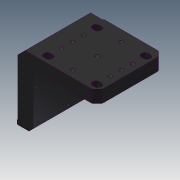
# Autodesk Inventor part: J003053
Saved by Autodesk Inventor 2015 SP1 (Build 190203100, 203)
## iProperties
Created: 2015-01-06
Material: ALUMINUM, 6061-T651
Vendor: HHMI: JFRC - ID&F
Document SubType Name: Modeling
Designer: ARNOLDJ
Density: 2.7 g/cm^3
Mass: 325.965 g
Surface Area: 259.814 cm^2
Volume: 120.728 cm^3
Description: MBS CONN LINK
Project: P-201804
Appearance: Rubber - Black
Part Number: J003053
RuleStatus: InUse
AfterDocSave0: file://Part Number Cleaner
LAB/DEPT: SVOBODA (LAB)
REQUESTING SCIENTIST: SOFRONIEW, NICK
SURFACE ROUGHNESS: 63 Ra
DESIGN DEPARTMENT: HHMI: JRC - ID&F
SPECIAL FINISH: ANODIZE PER MIL-A-8625F, TYPE II, CLASS 2 (BLACK)
ALTERED ITEM PART NUMBER: N/A
ALTERED ITEM VENDOR: N/A
ALTERED ITEM DESCRIPTION: N/A
Revision Number: A
Autodesk Inventor part; units mm, degrees
ref_plane "YZ Plane" through (0, 0, 0) normal (1, 0, 0) x (0, 1, 0)
ref_plane "XZ Plane" through (0, 0, 0) normal (0, 1, 0) x (-1, 0, 0)
ref_plane "XY Plane" through (0, 0, 0) normal (0, 0, 1) x (1, 0, 0)
sketch "Sketch1" plane through (0, 0, 0) normal (0, 0, 1) x (1, 0, 0)
  line L0 (0, 45.1307) -> (0, -37.1551) projected
  line L1 (-35.56, 0) -> (35.56, 0) projected
  line L2 (25.4, 25.4) -> (25.4, -25.4) construction
  line L3 (25.4, -25.4) -> (-25.4, -25.4) construction
  line L4 (-25.4, -25.4) -> (-25.4, 25.4) construction
  line L5 (0, 33.3756) -> (15.875, 33.3756)
  line L6 (15.875, 33.3756) -> (15.875, -25.4)
  line L7 (15.875, -25.4) -> (0, -25.4)
  line L8 (0, -25.4) -> (0, 33.3756)
  point P0 (0, 0)
  point P1 (-25.4, 0)
  point P2 (0, -25.4)
  point P3 (0, 3.9878)
  dimension "d0" = 50.8
  dimension "d1" = 50.8
  dimension "d39" = 25.4
  dimension "d41" = 33.3756
  dimension "d76" = 15.875
  dimension "d77" = 0
  constraints: 14 end point, 3 midpoint, 2 parallel, 1 perpendicular, 1 vertical alignment
  measures "d0" distance of L4.end L2.start
  measures "d1" distance of L2.start L2.end
  measures "d39" distance between parallel lines of L1 L7
  measures "d41" distance between parallel lines of L1 L5
  measures "d76" distance of L5.start L5.end
  measures "d77" distance between parallel lines of L8 L0
extrude "Extrusion1" add sketch "Sketch1" along normal blind 39.0525 and the other way blind 28.8925
sketch "Sketch2" plane through (0, 33.3756, -28.8925) normal (0, 1, 0) x (1, 0, 0)
  line L0 (0, 0) -> (0, -67.945) projected
  line L1 (0, -67.945) -> (81.28, -67.945)
  line L2 (81.28, -67.945) -> (81.28, 0)
  line L3 (81.28, 0) -> (0, 0)
  line L4 (0, 0) -> (0, -67.945)
  dimension "d17" = 81.28
  dimension "d131" = 0
  constraints: 8 end point, 2 parallel, 1 horizontal, 1 perpendicular
  measures "d17" distance of L2.end L3.end
  measures "d131" distance from line of L0.start L3
extrude "Extrusion2" add sketch "Sketch2" along normal blind 12.7
sketch "Sketch4" plane through (0, 33.3756, -28.8925) normal (0, -1, 0) x (1, 0, 0)
  line L0 (81.28, 0) -> (15.875, 0) projected
  line L1 (81.28, 67.945) -> (81.28, 0) projected
  line L2 (71.4883, 0) -> (27.0383, 0)
  line L3 (27.0383, 0) -> (27.0383, 3.937)
  line L4 (27.0383, 3.937) -> (71.4883, 3.937)
  line L5 (-17.272, 28.8925) -> (103.632, 28.8925) projected
  line L6 (71.4883, 3.937) -> (71.4883, 0)
  line L7 (0, 90.043) -> (0, -64.643) projected
  line L8 (49.2633, 3.937) -> (49.2633, 0) construction
  line L9 (15.875, 67.945) -> (15.875, 0) projected
  point P0 (0, 28.8925)
  point P1 (0, -42.545)
  dimension "d64" = 24.9555
  dimension "d65" = 44.45
  dimension "d67" = 49.2633
  dimension "d80" = 11.1633
  constraints: 10 end point, 2 midpoint, 2 perpendicular, 1 horizontal, 1 parallel, 1 other
  measures "d64" distance between parallel lines of L4 L5
  measures "d65" distance of L3.end L4.end
  measures "d67" distance between parallel lines of L8 L7
  measures "d80" distance between parallel lines of L9 L3
extrude "Extrusion4" add sketch "Sketch4" along normal blind 2.54 contours L0 L3 L4 L6
sketch "Sketch6" plane through (0, 46.0756, -28.8925) normal (0, 1, 0) x (1, 0, 0)
  line L0 (74.1538, -60.937) -> (24.1538, -60.937)
  line L1 (24.1538, -60.937) -> (24.1538, -10.937)
  line L2 (24.1538, -10.937) -> (74.1538, -10.937)
  line L3 (74.1538, -10.937) -> (74.1538, -60.937)
  line L4 (24.1538, -35.937) -> (74.1538, -35.937) construction
  line L5 (49.1538, -10.937) -> (49.1538, -60.937) construction
  line L6 (27.0383, -3.937) -> (71.4883, -3.937) construction
  line L7 (0, 13.589) -> (0, -81.534) construction
  line L8 (19.7088, -7.4445) -> (28.5988, -7.4445)
  line L9 (28.5988, -7.4445) -> (28.5988, -14.4295)
  line L10 (28.5988, -14.4295) -> (19.7088, -14.4295)
  line L11 (19.7088, -14.4295) -> (19.7088, -7.4445)
  line L12 (69.7088, -7.4445) -> (78.5988, -7.4445)
  line L13 (78.5988, -7.4445) -> (78.5988, -14.4295)
  line L14 (78.5988, -14.4295) -> (69.7088, -14.4295)
  line L15 (69.7088, -14.4295) -> (69.7088, -7.4445)
  line L16 (19.7088, -57.4445) -> (28.5988, -57.4445)
  line L17 (28.5988, -57.4445) -> (28.5988, -64.4295)
  line L18 (28.5988, -64.4295) -> (19.7088, -64.4295)
  line L19 (19.7088, -64.4295) -> (19.7088, -57.4445)
  line L20 (69.7088, -57.4445) -> (78.5988, -57.4445)
  line L21 (78.5988, -57.4445) -> (78.5988, -64.4295)
  line L22 (78.5988, -64.4295) -> (69.7088, -64.4295)
  line L23 (69.7088, -64.4295) -> (69.7088, -57.4445)
  line L24 (99.06, -28.8925) -> (-16.51, -28.8925) projected
  point P0 (0, -28.8925)
  point P1 (19.7088, -10.937)
  point P2 (24.1538, -7.4445)
  point P3 (69.7088, -10.937)
  point P4 (74.1538, -7.4445)
  point P5 (19.7088, -60.937)
  point P6 (24.1538, -57.4445)
  point P7 (69.7088, -60.937)
  point P8 (74.1538, -57.4445)
  point P9 (81.28, -3.937)
  point P10 (15.875, -3.937)
  dimension "d46" = 50
  dimension "d47" = 50
  dimension "d51" = 49.1538
  dimension "d52" = 6.985
  dimension "d53" = 8.89
  dimension "d54" = 6.985
  dimension "d62" = 17.9555
  dimension "d63" = 7
  constraints: 44 end point, 12 midpoint, 10 parallel, 6 equal length, 5 horizontal, 5 perpendicular, 4 coincident, 4 horizontal alignment, 4 vertical alignment
  measures "d46" distance of L2.end L0.start
  measures "d47" distance of L0.start L0.end
  measures "d51" distance between parallel lines of L5 L7
  measures "d52" distance of L10.end L8.start
  measures "d53" distance of L8.start L8.end
  measures "d54" distance of L20.end L21.end
  measures "d62" distance from line of L2.end L24
  measures "d63" distance between parallel lines of L6 L2
extrude "Extrusion6" cut sketch "Sketch6" against normal up to next contours L3 L20 L21 L22 L23 L0 | L0 L23 L20 L3 | L17 L18 L19 L16 L1 L0 | L0 L1 L16 L17 | L14 L15 L2 L3 | L3 L2 L15 L12 L13 L14 | L10 L11 L8 L9 L2 L1 | L1 L2 L9 L10
fillet "Fillet2" radius 3.175 16 edges at (28.5988, 39.7256, -14.463) (28.5988, 39.7256, -21.448) (19.7088, 39.7256, -21.448) (19.7088, 39.7256, -14.463) (28.5988, 39.7256, 28.552) (28.5988, 39.7256, 35.537) (19.7088, 39.7256, 35.537) (19.7088, 39.7256, 28.552) (69.7088, 39.7256, 35.537) (69.7088, 39.7256, 28.552) (78.5988, 39.7256, 28.552) (78.5988, 39.7256, 35.537) (69.7088, 39.7256, -14.463) (69.7088, 39.7256, -21.448) (78.5988, 39.7256, -21.448) (78.5988, 39.7256, -14.463)
sketch "Sketch8" plane through (0, 0, 0) normal (1, 0, 0) x (0, 1, 0)
  line L0 (16, 3.05) -> (-16, 3.05) construction
  line L1 (-16, 3.05) -> (-16, 35.05) construction
  line L2 (-16, 35.05) -> (16, 35.05) construction
  line L3 (16, 35.05) -> (16, 3.05) construction
  point P0 (0, 0)
  dimension "d81" = 32
  dimension "d82" = 32
  dimension "d84" = 35.05
  dimension "d85" = 16
  constraints: 8 end point, 2 parallel, 1 horizontal, 1 perpendicular
  measures "d81" distance of L2.end L0.start
  measures "d82" distance of L0.start L0.end
  measures "d84" distance from line of point (0, 0) L2
  measures "d85" distance from line of point (0, 0) L1
hole "Hole3" at (0, 16, 3.05) at (0, 16, 35.05) at (0, -16, 35.05) at (0, -16, 3.05) direction (1, 0, 0) diameter 2.4638 end through all
sketch "Sketch9" plane through (0, 0, 0) normal (1, 0, 0) x (0, 1, 0)
  line L0 (17.905, -4.76) -> (14.095, -4.76)
  line L1 (14.095, -4.76) -> (14.095, -0.95)
  line L2 (14.095, -0.95) -> (17.905, -0.95)
  line L3 (17.905, -0.95) -> (17.905, -4.76)
  line L4 (-20, 38.455) -> (-23.81, 38.455)
  line L5 (-23.81, -0.355) -> (-20, -0.355)
  line L6 (-20, 3.455) -> (-23.81, 3.455)
  line L7 (-20, 34.645) -> (-23.81, 34.645)
  line L8 (-20, -0.355) -> (-20, 3.455)
  line L9 (-20, 34.645) -> (-20, 38.455) construction
  line L10 (-23.81, 38.455) -> (-23.81, 34.645)
  line L11 (-23.81, 3.455) -> (-23.81, -0.355)
  line L12 (-20, 1.55) -> (-23.81, 1.55) construction
  line L13 (-20, 36.55) -> (-23.81, 36.55) construction
  line L14 (0, 0) -> (34.4542, 0) construction
  line L15 (0, 0) -> (35.5729, 0) construction
  line L16 (-35.6866, 0) -> (47.4495, 0) construction
  line L17 (16, -0.95) -> (16, -4.76) construction
  line L18 (-14.095, -0.95) -> (-17.905, -0.95)
  line L19 (-17.905, -0.95) -> (-17.905, -4.76)
  line L20 (-17.905, -4.76) -> (-14.095, -4.76)
  line L21 (-14.095, -4.76) -> (-14.095, -0.95)
  line L22 (-16, -0.95) -> (-16, -4.76) construction
  line L23 (-20, 34.645) -> (-20, 38.455)
  dimension "d94" = 3.81
  dimension "d95" = 3.81
  dimension "d97" = 3.81
  dimension "d103" = 3.81
  dimension "d104" = 3.81
  dimension "d105" = 3.81
  dimension "d106" = 0
  dimension "d107" = 20
  dimension "d109" = 36.55
  dimension "d110" = 16
  dimension "d112" = 16
  dimension "d113" = 3.81
  dimension "d114" = 3.81
  dimension "d116" = 2.095
  dimension "d132" = 35
  dimension "d133" = 39.405
  dimension "d134" = 39.405
  constraints: 46 end point, 9 parallel, 9 perpendicular, 8 midpoint, 4 horizontal, 1 point on line
  measures "d94" distance of L2.end L0.start
  measures "d95" distance of L1.end L2.end
  measures "d97" distance of L5.start L5.end
  measures "d103" distance of L6.end L5.start
  measures "d104" distance of L7.start L7.end
  measures "d105" distance of L4.end L7.end
  measures "d106" distance between parallel lines of L9 L8
  measures "d107" distance from line of L9 L14.start
  measures "d109" distance between parallel lines of L16 L13
  measures "d110" distance from line of L14.start L17
  measures "d112" distance from line of L14.start L22
  measures "d113" distance of L20.end L18.start
  measures "d114" distance of L19.end L20.end
  measures "d116" distance between parallel lines of L8 L19
  measures "d132" distance between parallel lines of L13 L12
  measures "d133" distance between parallel lines of L4 L2
  measures "d134" distance between parallel lines of L4 L18
extrude "Extrusion7" add sketch "Sketch9" against normal blind 1.27
sketch "Sketch10" plane through (0, -25.4, -28.8925) normal (-1, 0, 0) x (0, 0, 1)
  line L0 (25.7175, 71.4756) -> (65.0875, 71.4756)
  line L1 (65.0875, 71.4756) -> (65.0875, 46.0756)
  line L2 (65.0875, 46.0756) -> (25.7175, 46.0756)
  line L3 (25.7175, 46.0756) -> (25.7175, 71.4756)
  line L4 (67.945, 71.4756) -> (0, 71.4756) projected
  point P0 (28.8925, 25.4)
  dimension "d117" = 0
  dimension "d120" = 25.4
  dimension "d137" = 36.195
  dimension "d138" = 3.175
  constraints: 8 end point, 2 parallel, 1 horizontal, 1 perpendicular
  measures "d117" distance between parallel lines of L4 L0
  measures "d120" distance of L2.end L0.start
  measures "d137" distance from line of L1 point (28.893, 25.4)
  measures "d138" distance from line of point (28.893, 25.4) L3
extrude "Extrusion8" cut sketch "Sketch10" against normal blind 7.62
chamfer "Chamfer3" distance 7.62 angle 45 2 edges at (0, 46.0756, -16.0338) (0, 46.0756, 37.6238)
fillet "Fillet4" radius 4.7625 2 edges at (3.81, 20.6756, 36.195) (3.81, 20.6756, -3.175)
chamfer "Chamfer4" distance 6.35 angle 45 1 edges at (15.875, -25.4, 5.08)
sketch "Sketch11" plane through (0, 46.0756, -28.8925) normal (0, 1, 0) x (1, 0, 0)
  line L0 (0, 13.589) -> (0, -81.534) projected
  line L1 (97.536, -28.8925) -> (-16.256, -28.8925) projected
  line L2 (75.4238, -64.4295) -> (72.8838, -64.4295) projected
  line L3 (72.8838, -57.4445) -> (75.4238, -57.4445) projected
  line L4 (75.4238, -14.4295) -> (72.8838, -14.4295) projected
  line L5 (72.8838, -7.4445) -> (75.4238, -7.4445) projected
  line L6 (22.8838, -7.4445) -> (25.4238, -7.4445) projected
  line L7 (25.4238, -14.4295) -> (22.8838, -14.4295) projected
  line L8 (22.8838, -57.4445) -> (25.4238, -57.4445) projected
  line L9 (25.4238, -64.4295) -> (22.8838, -64.4295) projected
  line L10 (72.8838, -64.4295) -> (75.4238, -64.4295) construction
  line L11 (74.1538, -64.4295) -> (74.1538, -57.4445) construction
  line L12 (22.8838, -64.4295) -> (25.4238, -64.4295) construction
  line L13 (24.1538, -64.4295) -> (24.1538, -57.4445) construction
  line L14 (25.4238, -57.4445) -> (22.8838, -57.4445) construction
  line L15 (72.8838, -14.4295) -> (75.4238, -14.4295) construction
  line L16 (74.1538, -14.4295) -> (74.1538, -7.4445) construction
  line L17 (22.8838, -14.4295) -> (25.4238, -14.4295) construction
  line L18 (24.1538, -14.4295) -> (24.1538, -7.4445) construction
  line L19 (74.1538, -60.937) -> (24.1538, -60.937) construction
  line L20 (74.1538, -10.937) -> (24.1538, -10.937) construction
  line L21 (74.1538, -57.4445) -> (74.1538, -14.4295) construction
  line L22 (24.1538, -57.4445) -> (24.1538, -14.4295) construction
  line L23 (74.1538, -35.937) -> (24.1538, -35.937) construction
  circle A0 centre (74.1538, -60.937) radius 6.5 construction
  circle A1 centre (74.1538, -47.367) radius 5.8 construction
  point P0 (0, -28.8925)
  point P1 (49.1538, -60.937)
  point P2 (49.1538, -10.937)
  point P3 (74.1538, -24.507)
  point P4 (24.1538, -24.507)
  point P5 (24.1538, -47.367)
  point P6 (49.1538, -35.937)
  dimension "d145" = 11.43
  dimension "d146" = 11.43
  dimension "d147" = 11.43
  dimension "d148" = 11.43
  dimension "d149" = 13
  dimension "d150" = 11.6
  constraints: 18 end point, 17 midpoint, 4 coincident, 4 point on line, 2 centre point, 2 perpendicular
  measures "d145" distance from line of point (74.154, -47.367) L23
  measures "d146" distance from line of point (24.154, -47.367) L23
  measures "d147" distance from line of point (74.154, -24.507) L23
  measures "d148" distance from line of point (24.154, -24.507) L23
  measures "d149" diameter of A0
  measures "d150" diameter of A1
hole "Hole4" at (74.1538, 46.0756, 18.4745) at (74.1538, 46.0756, 7.0445) at (74.1538, 46.0756, -4.3855) at (49.1538, 46.0756, -17.9555) at (49.1538, 46.0756, 7.0445) at (49.1538, 46.0756, 32.0445) at (24.1538, 46.0756, 18.4745) at (24.1538, 46.0756, 7.0445) at (24.1538, 46.0756, -4.3855) direction (0, -1, 0) diameter 4.1402 end through all
fillet "Fillet5" radius 3.175 2 edges at (4.7625, -25.4, 39.0525) (4.7625, -25.4, -28.8925)
chamfer "Chamfer5" distance 5.08 angle 45 2 edges at (81.28, 39.7256, -28.8925) (81.28, 39.7256, 39.0525)
fillet "Fillet7" radius 3.175 2 edges at (81.28, 39.7256, 33.9725) (81.28, 39.7256, -23.8125)
sketch "Sketch12" plane through (0, 0, -28.8925) normal (0, 0, -1) x (-1, 0, 0)
  line L0 (0, -39.6951) -> (0, 60.3707) projected
  line L1 (-97.79, 0) -> (17.78, 0) projected
  line L2 (-9.525, -25.4) -> (0, -25.4) projected
  line L3 (-7.62, 46.0756) -> (-74.8849, 46.0756) projected
  line L4 (-1.016, 46.0756) -> (-20.066, 46.0756)
  line L5 (-20.066, 46.0756) -> (-20.066, -25.4)
  line L6 (-20.066, -25.4) -> (-1.016, -25.4)
  line L7 (-1.016, -25.4) -> (-1.016, 46.0756)
  line L8 (-7.62, 46.0756) -> (0, 38.4556) projected
  line L9 (0, 38.4556) -> (-1.016, 38.4556)
  line L10 (-1.016, 38.4556) -> (-1.016, 39.4716)
  line L11 (-1.016, 39.4716) -> (0, 39.4716)
  line L12 (0, 39.4716) -> (0, 38.4556)
  point P0 (0, 0)
  point P1 (-10.016, 42.9006)
  point P2 (-10.016, 12.9006)
  point P3 (-10.016, -17.0994)
  dimension "d158" = 19.05
  dimension "d159" = 0
  dimension "d160" = 1.016
  dimension "d161" = 0
  dimension "d164" = 30
  dimension "d165" = 71.4756
  dimension "d166" = 9
  dimension "d167" = 30
  dimension "d168" = 3.175
  constraints: 16 end point, 4 parallel, 2 horizontal, 2 perpendicular, 2 point on line, 2 vertical alignment
  measures "d158" distance of L4.start L4.end
  measures "d159" distance between parallel lines of L4 L3
  measures "d160" distance between parallel lines of L0 L7
  measures "d161" distance between parallel lines of L2 L6
  measures "d164" distance of point (-10.016, 12.901) point (-10.016, -17.099)
  measures "d165" distance of L4.end L5.end
  measures "d166" distance from line of point (-10.016, -17.099) L7
  measures "d167" distance of point (-10.016, 12.901) point (-10.016, 42.901)
  measures "d168" distance from line of point (-10.016, 42.901) L4
extrude "Extrusion9" cut sketch "Sketch12" against normal blind 1.016 contours L9 L7 L8 | L8 L4 L7 | L7 L1 L5 L3 L8 | L7 L2 L6 L5 L1
hole "Hole5" at (10.016, 42.9006, -28.8925) at (10.016, 12.9006, -28.8925) at (10.016, -17.0994, -28.8925) direction (0, 0, 1) diameter 2.4638 depth 8.89 tip angle 118
body "Solid1"
